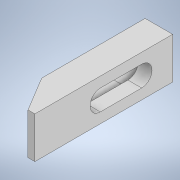
# Autodesk Inventor part: Lengueta 2 LRP
Saved by Autodesk Inventor 2020 (Build 240168000, 168)
## iProperties
Created: 2020-05-30
Part Number: Lengueta 2 LRP
Material: Genérico
Document SubType Name: Modeling
Designer: Pipi
Density: 1 g/cm^3
Appearance: Valor por defecto
Author: Pipi
Autodesk Inventor part; units mm, degrees
ref_plane "YZ Plane" through (0, 0, 0) normal (1, 0, 0) x (0, 1, 0)
ref_plane "XZ Plane" through (0, 0, 0) normal (0, 1, 0) x (-1, 0, 0)
ref_plane "XY Plane" through (0, 0, 0) normal (0, 0, 1) x (1, 0, 0)
sketch "Boceto1" plane through (0, 0, 0) normal (0, 1, 0) x (-1, 0, 0)
  line L0 (3.0387, 17.5812) -> (3.0387, -22.4188)
  line L1 (3.0387, -22.4188) -> (11.0387, -22.4188)
  line L2 (11.0387, -22.4188) -> (11.0387, 7.5812)
  line L3 (3.0387, 17.5812) -> (5.0387, 17.5812)
  line L4 (5.0387, 17.5812) -> (11.0387, 7.5812)
  point P0 (0, 0)
  dimension "d0" = 40
  dimension "d1" = 8
  dimension "d2" = 30
  dimension "d3" = 2
  constraints: 10 end point, 2 perpendicular, 1 horizontal, 1 vertical
  measures "d0" distance of L0.start L0.end
  measures "d1" distance of L0.end L1.end
  measures "d2" distance of L1.end L2.end
  measures "d3" distance of L0.start L3.end
extrude "Extrusión1" add sketch "Boceto1" along normal blind 12
sketch "Boceto2" plane through (-11.0387, 0, -22.4188) normal (-1, 0, 0) x (0, 0, 1)
  line L0 (0, 0) -> (0, 12) projected
  line L1 (30, 0) -> (30, 12) projected
  line L2 (0, 6) -> (30, 6)
  line L3 (15, 6) -> (15, 9)
  line L4 (15, 9) -> (9, 9)
  line L5 (9, 9) -> (21, 9)
  line L6 (15, 3) -> (9, 3)
  line L7 (9, 3) -> (21, 3)
  line L8 (15, 6) -> (15, 11)
  line L9 (0, 12) -> (30, 12) projected
  line L10 (15, 11) -> (9, 11)
  line L11 (9, 11) -> (21, 11)
  line L12 (9, 1) -> (21, 1)
  arc A0 (9, 9) -> (9, 3) centre (9, 6) ccw
  arc A1 (21, 3) -> (21, 9) centre (21, 6) ccw
  arc A2 (21, 1) -> (21, 11) centre (21, 6) ccw
  arc A3 (9, 11) -> (9, 1) centre (9, 6) ccw
  dimension "d22" = 3
  dimension "d23" = 6
  dimension "d24" = 12
  dimension "d25" = 5
  dimension "d26" = 6
  dimension "d27" = 12
  dimension "d28" = 3
  dimension "d29" = 3
  dimension "d30" = 5
  dimension "d31" = 5
  constraints: 20 end point, 8 point on circle, 5 symmetric about line, 4 centre point, 3 midpoint, 3 perpendicular, 3 point on line, 1 vertical
  measures "d22" distance of L3.start L3.end
  measures "d23" distance of L3.end L4.end
  measures "d24" distance of L4.end L5.end
  measures "d25" distance of L3.start L8.end
  measures "d26" distance of L8.end L10.end
  measures "d27" distance of L10.end L11.end
  measures "d28" radius of A0
  measures "d29" radius of A1
  measures "d30" radius of A2
  measures "d31" radius of A3
extrude "Extrusión4" cut sketch "Boceto2" against normal blind 44 contours A0 L4 L3 L2 | L2 A1 L7 L6 A0 | L3 L5 A1 L2
extrude "Extrusión5" cut sketch "Boceto2" against normal blind 4 contours A3 L10 L8 L4 A0 L2 | L2 A0 L6 L7 A1 A2 L12 A3 | L11 A2 L2 A1 L5 L8
